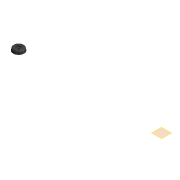
# Autodesk Inventor part: foot
Saved by Autodesk Inventor 2014 (Build 180170000, 170)
## iProperties
Created: 2016-03-30
Part Number: foot
Material: Rubber
Document SubType Name: Modeling
Designer: admin
Density: 0.93 g/cm^3
Appearance: Rubber - Black - Version 1.1
Author: admin
Autodesk Inventor part; units mm, degrees
ref_plane "YZ Plane" through (0, 0, 0) normal (1, 0, 0) x (0, 1, 0)
ref_plane "XZ Plane" through (0, 0, 0) normal (0, 1, 0) x (-1, 0, 0)
ref_plane "XY Plane" through (0, 0, 0) normal (0, 0, 1) x (1, 0, 0)
ref_plane "Work Plane1" through (0, 0, 0) normal (0, 0, 1) x (1, 0, 0)
sketch "Sketch1" plane through (0, 0, 0) normal (0, 0, 1) x (1, 0, 0)
  circle A0 centre (-150, 86.6025) radius 13 projected
  circle A1 centre (0, -173.2051) radius 13 projected
  circle A2 centre (0, -173.2051) radius 11.5
  circle A3 centre (-150, 86.6025) radius 11.5
  circle A4 centre (150, 86.6025) radius 11.5
  circle A5 centre (-150, 86.6025) radius 13 projected
  point P0 (0, 0)
  dimension "d0" = 23
  dimension "d1" = 23
  dimension "d2" = 23
  constraints: 3 centre point, 2 coincident
  measures "d0" diameter of A2
  measures "d1" diameter of A3
  measures "d2" diameter of A4
extrude "Extrusion1" add sketch "Sketch1" along normal blind 6 draft -10 contours A3
fillet "Fillet1" radius 2 1 edges at (-160.442, 86.6025, 6)
sketch "Sketch2" plane through (-150, 86.6025, 6) normal (0, 0, 1) x (1, 0, 0)
  circle A0 centre (0, 0) radius 8.7638 projected
  circle A1 centre (0, 0) radius 5
  point P0 (150, -86.6025)
  dimension "d6" = 10
  constraints: 1 centre point, 1 coincident
  measures "d6" diameter of A1
extrude "Extrusion2" cut sketch "Sketch2" against normal blind 3 contours A1
sketch "Sketch3" plane through (-150, 86.6025, 3) normal (0, 0, 1) x (1, 0, 0)
  circle A0 centre (0, 0) radius 5 projected
  circle A1 centre (0, 0) radius 2
  point P0 (150, -86.6025)
  dimension "d9" = 4
  constraints: 1 centre point, 1 coincident
  measures "d9" diameter of A1
extrude "Extrusion3" cut sketch "Sketch3" against normal blind 3 contours A1
sketch "Sketch4" plane through (-150, 86.6025, 6) normal (0, 0, 1) x (1, 0, 0)
  circle A0 centre (0, 0) radius 5 projected
  circle A1 centre (0, 0) radius 8.7638 projected
  circle A2 centre (0, 0) radius 8
  point P0 (150, -86.6025)
  dimension "d12" = 16
  constraints: 1 centre point, 1 coincident
  measures "d12" diameter of A2
extrude "Extrusion4" cut sketch "Sketch4" against normal blind 0.5 contours A2
body "Solid1"
